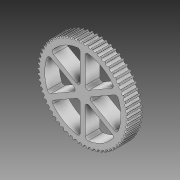
# Autodesk Inventor part: Timing Pulley Generator
Saved by Autodesk Inventor 2022 (Build 260153000, 153)
## iProperties
Created: 2022-01-03
Part Number: Timing Pulley Generator
Material: Generic
Document SubType Name: Modeling
Density: 1 g/cm^3
Appearance: Default
Part Number: Timing Pulley Generator HTD
Autodesk Inventor part; units mm, degrees
ref_plane "YZ Plane" through (0, 0, 0) normal (1, 0, 0) x (0, 1, 0)
ref_plane "XZ Plane" through (0, 0, 0) normal (0, 1, 0) x (-1, 0, 0)
ref_plane "XY Plane" through (0, 0, 0) normal (0, 0, 1) x (1, 0, 0)
sketch "Sketch1" plane through (0, 0, 0) normal (0, 0, 1) x (1, 0, 0)
  circle A0 centre (0, 0) radius 28.6479
  dimension "d0" = 57.2958
  constraints: 1 centre point, 1 coincident
  measures "d0" diameter of A0
extrude "Base" add sketch "Sketch1" along normal mid plane 9
sketch "Sketch2" plane through (0, 0, 4.5) normal (0, 0, 1) x (1, 0, 0)
  arc A0 (0.541, 28.0677) -> (0, 28.0729) centre (0, 0) ccw
  arc A1 (0.9192, 27.4491) -> (0.541, 28.0677) centre (0.5327, 27.6378) ccw
  arc A2 (0.9192, 27.4491) -> (0.9271, 26.0544) centre (2.3314, 26.7598) ccw
  circle A3 centre (0, 0) radius 28.6479 construction
  line L0 (0, 0) -> (0, 28.0729) construction
  line L1 (-12.5179, 29.3432) -> (15.5165, 27.874) construction
  arc A4 (1.4993, 28.6086) -> (0, 28.6479) centre (0, 0) ccw
  line L2 (0, 28.0729) -> (0, 28.6479)
  line L3 (0, 0) -> (1.4993, 28.6086)
  line L4 (0.9271, 26.0544) -> (1.3476, 25.7139)
  dimension "d3" = 0.43
  dimension "d4" = 1.5715
  dimension "d5" = 0.575
  dimension "d6" = 2.6175
  dimension "d13" = 3
  dimension "d15" = 0.5411
  dimension "d17" = 0.5411
  dimension "d18" = 54
  constraints: 10 end point, 10 point on circle, 4 centre point, 3 tangent, 2 coincident, 2 vertical, 2 vertical alignment, 1 equal length, 1 midpoint, 1 point on line
  measures "d3" radius of A1
  measures "d4" radius of A2
  measures "d5" distance of L0.end L2.end
  measures "d6" distance of L3.end L4.start
  measures "d13" angle of L0 L3
  measures "d17" distance of L4.start L4.end
  measures "d18" angle of L3 L4
extrude "HTD .5 tooth" [suppressed]
mirror "HTD tooth" [suppressed]
pattern_circular "HTD profile" [suppressed]
fillet "HTD fillet" [suppressed]
pattern_circular "HTD teeth" [suppressed]
sketch "Sketch5" plane through (0, 0, 4.5) normal (0, 0, 1) x (1, 0, 0)
  circle A0 centre (0, 0) radius 28.6479 projected
  arc A1 (0.5418, 27.9547) -> (0.2308, 28.2709) centre (0.2283, 27.9575) ccw
  arc A2 (0.5544, 27.7458) -> (1.4125, 26.9512) centre (1.4603, 27.8635) ccw
  line L0 (0, 0) -> (0, 28.2719) construction
  line L1 (-12.6173, 29.3484) -> (15.6159, 27.8688) construction
  arc A3 (1.4993, 28.6086) -> (0, 28.6479) centre (0, 0) ccw
  line L2 (0, 28.2719) -> (0, 28.6479)
  line L3 (0, 0) -> (1.4993, 28.6086)
  arc A4 (0.5418, 27.9547) -> (0.5544, 27.7458) centre (2.0617, 27.9416) ccw
  arc A5 (0.2308, 28.2709) -> (0, 28.2719) centre (0, 0) ccw
  arc A6 (2.1081, 28.5702) -> (1.4993, 28.6086) centre (0, 0) ccw construction
  line L4 (2.0617, 27.9416) -> (0, 0) construction
  line L5 (3.6005, 28.4207) -> (3.4093, 26.9121) construction
  point P0 (1.4993, 28.6086)
  dimension "d35" = 0.3135
  dimension "d36" = 0.9135
  dimension "d37" = 0.376
  dimension "d39" = 3
  dimension "d52" = 1.52
  dimension "d54" = 0.61
  dimension "d61" = 1.6597
  dimension "d62" = 1.5207
  dimension "d63" = 3
  constraints: 13 end point, 12 point on circle, 6 centre point, 4 coincident, 3 point on line, 3 tangent, 2 vertical, 1 equal length, 1 line through centre, 1 midpoint, 6 other
  measures "d35" radius of A1
  measures "d36" radius of A2
  measures "d37" distance of L0.end L2.end
  measures "d39" angle of L0 L3
  measures "d52" radius of A4
  measures "d61" distance of L3.end A2.end
  measures "d62" distance of L5.start L5.end
  measures "d63" angle of L5 L4
extrude "GT2 .5 tooth" cut sketch "Sketch5" against normal through all contours L3 A2 A4 A1 A5 L2 A0 picked at (1.3721, 27.5155)
mirror "GT2 tooth" about plane through (0, 0, 0) normal (1, 0, 0) of "GT2 .5 tooth"
pattern_circular "Circular Pattern3" count 60 over 360 about axis through (0, 0, -10) along (0, 0, 1) of "GT2 .5 tooth", "GT2 tooth"
sketch "Sketch6" plane through (0, 0, 4.5) normal (0, 0, 1) x (1, 0, 0)
  circle A0 centre (0, 0) radius 23.8125
  circle A1 centre (0, 0) radius 4.7625
  line L0 (0, 0) -> (0, 23.8125) construction
  line L1 (1.5875, 0) -> (1.5875, 23.8125)
  line L2 (-1.5875, 23.8125) -> (-1.5875, 0)
  arc A2 (-1.5875, 0) -> (1.5875, 0) centre (0, 0) ccw
  arc A3 (1.5875, 23.8125) -> (-1.5875, 23.8125) centre (0, 23.8125) ccw
  line L3 (0, 0) -> (20.6222, 11.9063) construction
  line L4 (0.7938, -1.3748) -> (21.416, 10.5314)
  line L5 (19.8285, 13.2811) -> (-0.7938, 1.3748)
  line L6 (0, 0) -> (20.6222, -11.9062) construction
  line L7 (-0.7937, -1.3748) -> (19.8285, -13.2811)
  line L8 (21.416, -10.5314) -> (0.7937, 1.3748)
  line L9 (0, 0) -> (0, -23.8125) construction
  line L10 (-1.5875, 0) -> (-1.5875, -23.8125)
  line L11 (1.5875, -23.8125) -> (1.5875, 0)
  line L12 (0, 0) -> (-20.6222, -11.9063) construction
  line L13 (-0.7938, 1.3748) -> (-21.416, -10.5314)
  line L14 (-19.8285, -13.2811) -> (0.7938, -1.3748)
  line L15 (0, 0) -> (-20.6222, 11.9062) construction
  line L16 (0.7937, 1.3748) -> (-19.8285, 13.2811)
  line L17 (-21.416, 10.5314) -> (-0.7937, -1.3748)
  point P0 (0, 11.9062)
  point P1 (-4.6823, 0.8702)
  point P2 (-21.3701, 10.5049)
  point P3 (-21.3701, -10.5049)
  point P4 (-4.6823, -0.8702)
  point P5 (-3.0948, -3.6199)
  point P6 (-19.7826, -13.2546)
  point P7 (-1.5875, -23.7595)
  point P8 (-1.5875, -4.4901)
  point P9 (1.5875, -4.4901)
  point P10 (1.5875, -23.7595)
  point P11 (19.7826, -13.2546)
  point P12 (3.0948, -3.6199)
  point P13 (4.6823, -0.8702)
  point P14 (21.3701, -10.5049)
  point P15 (21.3701, 10.5049)
  point P16 (4.6823, 0.8702)
  point P17 (3.0948, 3.6199)
  point P18 (19.7826, 13.2546)
  point P19 (1.5875, 23.7595)
  point P20 (1.5875, 4.4901)
  point P21 (-19.7826, 13.2546)
  point P22 (-3.0948, 3.6199)
  point P23 (-1.5875, 4.4901)
  point P24 (-1.5875, 23.7595)
  dimension "d65" = 47.625
  dimension "d66" = 9.525
  dimension "d67" = 3.175
  dimension "d70" = 360
  constraints: 48 end point, 4 point on circle, 4 tangent, 3 centre point, 2 coincident, 1 midpoint, 1 parallel, 1 vertical, 58 other
  measures "d66" diameter of A1
  measures "d67" diameter of A3
extrude "Extrusion5" cut sketch "Sketch6" against normal through all contours A0 L8 A1 L4 | L5 A1 L1 A0 | A0 L11 A1 L7 | L2 A1 L16 A0 | A0 L14 A1 L10 | L17 A1 L13 A0
fillet "Fillet3" radius 1.5875 24 edges at (4.6823, -0.8702, 0) (21.3701, -10.5049, 0) (21.3701, 10.5049, 0) (4.6823, 0.8702, 0) (-4.6823, 0.8702, 0) (-21.3701, 10.5049, 0) (-21.3701, -10.5049, 0) (-4.6823, -0.8702, 0) (3.0948, 3.6199, 0) (19.7826, 13.2546, 0) (1.5875, 23.7595, 0) (1.5875, 4.4901, 0) (1.5875, -4.4901, 0) (1.5875, -23.7595, 0) (19.7826, -13.2546, 0) (3.0948, -3.6199, 0) (-3.0948, -3.6199, 0) (-19.7826, -13.2546, 0) (-1.5875, -23.7595, 0) (-1.5875, -4.4901, 0) (-19.7826, 13.2546, 0) (-3.0948, 3.6199, 0) (-1.5875, 4.4901, 0) (-1.5875, 23.7595, 0)
equation "\"d0\" = Pitch_Diameter"
equation "\"d1\" = Width"
equation "\"d3\" = HTD_Root_Fillet_Rad"
equation "\"d6\" = HTD_Belt_Tooth_Height + HTD_Root_to_Pitch_Diameter - HTD_Subtractor"
equation "\"d17\" = d15"
equation "\"d8\" = Width"
equation "\"Pitch\" = 3"
equation "\"Width\" = 9"
equation "\"HTD_Root_Fillet_Rad\" = 0.43"
equation "\"HTD_Tooth_Rad\" = 1.49"
equation "\"HTD_Belt_Height\" = 3.8"
equation "\"HTD_Belt_Tooth_Height\" = 2.06"
equation "\"HTD_Root_to_Pitch_Diameter\" = -0.5 * HTD_Belt_Tooth_Height + 0.5 * HTD_Belt_Height"
equation "\"HTD_Subtractor\" = 0.3125"
equation "\"GT2_Root_Fillet_Rad\" = 0.25"
equation "\"GT2_Root_to_Pitch_Diameter\" = 0.63"
equation "\"GT2_Tooth_Rad\" = 0.85"
equation "\"GT2_Belt_Tooth_Height\" = 1.14"
equation "\"GT2_Belt_Height\" = 2.4"
equation "\"GT2_Middle_Rad\" = 1.52"
equation "\"GT2_Pitch_Offset\" = 0.61"
equation "\"GT2_Teeth_Adjusted\" = 0.6858"
equation "\"Pitch_Diameter\" = 57.29578"
body "Solid1"
